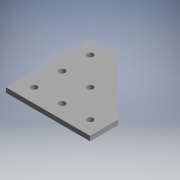
# Autodesk Inventor part: 4461
Saved by Autodesk Inventor 2017.3 (Build 213256000, 256)
## iProperties
Part Number: 4461
Material: Generic
Catalog Web Link: www.cadenas.de
Description: 4061, 4461, 4061-Black, 4461-Black-6 Hole 90 deg Joining Plate
Vendor: 8020
Document SubType Name: Modeling
Designer: partserver
Manufacturer: 8020
Mass: 62.4471 g
Surface Area: 232.854 cm^2
Volume: 62.4471 cm^3
Density: 1 g/cm^3
Appearance: PSOLRGB-191-191-191
Category: PARTsolutions
Company: 8020
Title: 4461
Author: Cadenas PARTsolutions
Comments: 6 Hole 90 deg Joining Plate
PSOL_IDENT_0: {$CADENAS_DATA\23d-libs\8020\inch\joining_plates\4061.prj},176 {VTYP=3D},{NB=4461},{LINA=4461},{NN=4
PSOL_IDENT_1: 061, 4461, 4061-Black, 4461-Black},{DATE=31.07.2020 09:21:18},{GEOMDATE=11.07.2017 15:23:36},{VERSIO
PSOL_IDENT_2: N=},{LINEID=20},{WBVAR=},{WBNUMERIC=}  {NB=4461},{LINA=4461},{KT=DUMMY},{PN=4461},{A=4.500},{B=1.500
PSOL_IDENT_3: },{F=0.328},{W=.370},{A1=0.7500},{C1=1.500},{C2=0.75},{D1=0.250},{COLOR=.75,.75,.75}
NB: 4461
NN: 4061, 4461, 4061-Black, 4461-Black
NT: 6 Hole 90 deg Joining Plate
NBSYN: $PN.
LINA: 4461
CATALOG: 80/20
PN: 4461
A: 4.5
B: 1.5
W: .370
SUPPLIER: 8020
ARTICLENO: 4461
BOMINFO: 4461
CREATOR: CADENAS GmbH
Autodesk Inventor part; units mm, degrees
ref_plane "YZ Plane" through (0, 0, 0) normal (1, 0, 0) x (0, 1, 0)
ref_plane "XZ Plane" through (0, 0, 0) normal (0, 1, 0) x (-1, 0, 0)
ref_plane "XY Plane" through (0, 0, 0) normal (0, 0, 1) x (1, 0, 0)
sketch "Sketch_1" plane through (0, 0, 0) normal (0, 0, 1) x (1, 0, 0)
  line L0 (-57.15, 38.1) -> (-57.15, 0)
  line L1 (-57.15, 0) -> (57.15, 0)
  line L2 (57.15, 0) -> (57.15, 114.3)
  line L3 (57.15, 114.3) -> (19.05, 114.3)
  line L4 (19.05, 114.3) -> (-57.15, 38.1)
  circle A0 centre (38.1, 19.05) radius 4.1656
  circle A1 centre (38.1, 57.15) radius 4.1656
  circle A2 centre (38.1, 95.25) radius 4.1656
  circle A3 centre (0, 19.05) radius 4.1656
  circle A4 centre (0, 57.15) radius 4.1656
  circle A5 centre (-38.1, 19.05) radius 4.1656
  constraints: 10 end point, 6 centre point
extrude "Extrusion1" add sketch "Sketch_1" along normal mid plane 6.35
body "Solid1"
